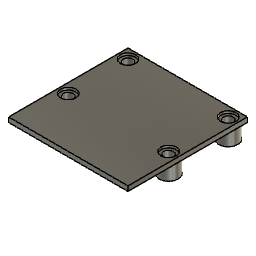
Attache caméra_PART2 (Autodesk Fusion 360 design; units mm, degrees)
Autodesk Fusion 360 part; units mm, degrees
sketch "Esquisse1" plane through (0, 0, 0) normal (0, 0, 1) x (1, 0, 0)
  line L0 (-12.5, 12.5) -> (12.5, 12.5)
  line L1 (12.5, 12.5) -> (12.5, -12.5)
  line L2 (12.5, -12.5) -> (-12.5, -12.5)
  line L3 (-12.5, -12.5) -> (-12.5, 12.5)
  circle A0 centre (-10.5, 10.5) radius 1
  circle A1 centre (10.5, 10.5) radius 1
  circle A2 centre (-10.5, -2) radius 1
  circle A3 centre (10.5, -2) radius 1
  dimension "d1" = 25
  dimension "d2" = 25
  dimension "d3" = 12.5
  dimension "d4" = 12.5
  dimension "d5" = 21
  dimension "d6" = 2
  dimension "d7" = 2
  dimension "d8" = 2
  dimension "d9" = 2
  dimension "d10" = 2
  dimension "d11" = 12.5
  dimension "d12" = 12.5
  dimension "d13" = 21
  dimension "d14" = 2
  dimension "d15" = 2
  dimension "d16" = 2
  dimension "d17" = 2
  constraint horizontal L0
  constraint vertical L1
  constraint horizontal L2
  constraint vertical L3
  measures "d1" distance of L0.start L0.end
  measures "d2" distance of L0.start L2.end
  measures "d3" distance of origin L0
  measures "d4" distance of origin L3
  measures "d5" distance of A0.centre A1.centre
  measures "d6" distance of L1 A1.centre
  measures "d7" distance of L0 A0.centre
  measures "d8" diameter of A0
  measures "d9" diameter of A1
  measures "d10" distance of L0 A1.centre
  measures "d11" vertical distance of A1.centre A3.centre
  measures "d12" vertical distance of A0.centre A2.centre
  measures "d13" distance of A2.centre A3.centre
  measures "d14" distance of L1 A3.centre
  measures "d15" distance of L3 A2.centre
  measures "d16" diameter of A3
  measures "d17" diameter of A2
extrude "Extrusion1" add sketch "Esquisse1" along normal blind 1
sketch "Esquisse2" plane through (0, 0, 0) normal (0, 0, -1) x (1, 0, 0)
  circle A0 centre (-10.5, 2) radius 1
  circle A1 centre (10.5, -10.5) radius 1
  circle A2 centre (10.5, 2) radius 1
  circle A3 centre (-10.5, -10.5) radius 1
  line L0 (12.5, 12.5) -> (-12.5, 12.5)
  line L1 (-12.5, 12.5) -> (-12.5, -12.5)
  line L2 (-12.5, -12.5) -> (12.5, -12.5)
  line L3 (12.5, -12.5) -> (12.5, 12.5)
  circle A4 centre (-10.5, -10.5) radius 2
  circle A5 centre (-10.5, 2) radius 2
  circle A6 centre (10.5, 2) radius 2
  circle A7 centre (10.5, -10.5) radius 2
  circle A8 centre (-10.5, 2) radius 1
  circle A9 centre (10.5, 2) radius 1
  circle A10 centre (-10.5, -10.5) radius 1
  circle A11 centre (10.5, -10.5) radius 1
  dimension "d20" = 4
  dimension "d21" = 4
  dimension "d22" = 4
  dimension "d23" = 4
  dimension "d26" = 2
  constraint concentric A3 A4
  constraint concentric A0 A5
  constraint concentric A2 A6
  constraint concentric A1 A7
  constraint concentric A5 A8
  constraint concentric A6 A9
  constraint concentric A4 A10
  constraint concentric A7 A11
  measures "d20" diameter of A5
  measures "d21" diameter of A6
  measures "d22" diameter of A7
  measures "d23" diameter of A4
  measures "d26" diameter of A8
extrude "Extrusion2" add sketch "Esquisse2" along normal blind 3 contours A5 | A6 | A7 | A4
sketch "Esquisse3" plane through (0, 0, 1) normal (0, 0, 1) x (-1, 0, 0)
  circle A0 centre (10.5, 2) radius 1
  circle A1 centre (-10.5, 2) radius 1
  circle A2 centre (-10.5, -10.5) radius 1
  circle A3 centre (10.5, -10.5) radius 1
  line L0 (12.5, 12.5) -> (-12.5, 12.5)
  line L1 (-12.5, 12.5) -> (-12.5, -12.5)
  line L2 (-12.5, -12.5) -> (12.5, -12.5)
  line L3 (12.5, -12.5) -> (12.5, 12.5)
  circle A4 centre (10.5, -10.5) radius 1.6
  circle A5 centre (-10.5, -10.5) radius 1.6
  circle A6 centre (-10.5, 2) radius 1.6
  circle A7 centre (10.5, 2) radius 1.6
  dimension "d27" = 3.2
  dimension "d28" = 3.2
  dimension "d29" = 3.2
  dimension "d30" = 3.2
  constraint concentric A3 A4
  constraint concentric A2 A5
  constraint concentric A1 A6
  constraint concentric A0 A7
  measures "d27" diameter of A4
  measures "d28" diameter of A5
  measures "d29" diameter of A6
  measures "d30" diameter of A7
extrude "Extrusion3" cut sketch "Esquisse3" against normal blind 0.5 contours A4 | A5 | A6 | A7
